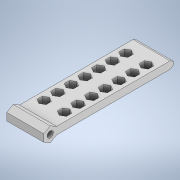
# Autodesk Inventor part: HexFlipper
Saved by Autodesk Inventor 2020 (Build 240168000, 168)
## iProperties
Created: 2023-12-22
Part Number: HexFlipper
Material: Generic
Document SubType Name: Modeling
Designer: smz3rm
Density: 1 g/cm^3
Appearance: Default
FlipperRodLength: 63.072 mm
Author: smz3rm
Autodesk Inventor part; units mm, degrees
ref_plane "YZ Plane" through (0, 0, 0) normal (1, 0, 0) x (0, 1, 0)
ref_plane "XZ Plane" through (0, 0, 0) normal (0, 1, 0) x (-1, 0, 0)
ref_plane "XY Plane" through (0, 0, 0) normal (0, 0, 1) x (1, 0, 0)
sketch "Sketch1" plane through (0, 0, 0) normal (1, 0, 0) x (0, 1, 0)
  line L0 (2, 35) -> (-2, 35)
  line L1 (-2, 35) -> (-2, -35)
  line L2 (-2, -35) -> (2, -35)
  line L3 (2, -35) -> (2, 35)
  line L4 (2, 35) -> (-2, -35) construction
  line L5 (-2, 35) -> (2, -35) construction
  line L6 (-1, -35) -> (-2, -33.2679)
  line L7 (-2, -33.2679) -> (-1, -31.5359)
  line L8 (-1, -31.5359) -> (1, -31.5359)
  line L9 (1, -31.5359) -> (2, -33.2679)
  line L10 (2, -33.2679) -> (1, -35)
  line L11 (1, -35) -> (-1, -35)
  line L12 (4, 31.5359) -> (2, 28.0718)
  line L13 (2, 28.0718) -> (-2, 28.0718)
  line L14 (-2, 28.0718) -> (-4, 31.5359)
  line L15 (-4, 31.5359) -> (-2, 35)
  line L16 (-2, 35) -> (2, 35)
  line L17 (2, 35) -> (4, 31.5359)
  circle A0 centre (0, 31.5359) radius 1.65
  point P0 (0, 0)
  point P1 (0, -33.2679)
  dimension "d0" = 4
  dimension "d1" = 70
  dimension "d2" = 3.3
  constraints: 36 end point, 4 point on line, 2 midpoint, 2 parallel, 1 centre point, 1 coincident, 1 horizontal, 1 perpendicular, 26 other
  measures "d0" distance of L2.end L1.end
  measures "d1" distance of L1.end L0.end
  measures "d2" diameter of A0
extrude "Extrusion1" add sketch "Sketch1" along normal mid plane 20 contours L3 L13 L1 L0 | L17 L12 L3 | L1 L14 L15 | L3 L9 L8 L7 L1 L13 | L10 L2 L6 L7 L8 L9
ref_plane "Work Plane1" through (-10, 2, 28.0718) normal (0, 0, -1) x (1, 0, 0)
sketch "Sketch2" plane through (-10, -1, -35) normal (0, 0, -1) x (-1, 0, 0)
  line L0 (-20, 2) -> (0, 2) projected
  line L1 (0, 0) -> (-20, 0) projected
  line L2 (-10, 2) -> (-10, 0)
  circle A0 centre (-10, 1) radius 1
  point P0 (-10, 1)
  dimension "d5" = 2
  constraints: 3 midpoint, 2 end point, 1 centre point, 1 vertical
  measures "d5" diameter of A0
extrude "Extrusion2" cut sketch "Sketch2" against normal up to surface (63.0718 mm away)
sketch "Sketch3" plane through (-10, 2, 28.0718) normal (0, 1, 0) x (1, 0, 0)
  line L0 (9, 63.0718) -> (9, 0) projected
  line L1 (11, 63.0718) -> (11, 0) projected
  line L2 (0, 0) -> (0, 61.3397) projected
  line L3 (0, 0) -> (20, 0) projected
  line L4 (20, 61.3397) -> (20, 0) projected
  line L5 (0, 61.3397) -> (20, 61.3397) projected
  line L6 (2, 2) -> (2, 59.3397)
  line L7 (2, 59.3397) -> (18, 59.3397)
  line L8 (18, 59.3397) -> (18, 2)
  line L9 (18, 2) -> (2, 2)
  line L10 (7, 63.0718) -> (7, 0)
  line L11 (13, 63.0718) -> (13, 0)
  line L12 (2, 51.5924) -> (2, 54.4791)
  line L13 (2, 54.4791) -> (4.5, 55.9225)
  line L14 (4.5, 55.9225) -> (7, 54.4791)
  line L15 (7, 54.4791) -> (7, 51.5924)
  line L16 (7, 51.5924) -> (4.5, 50.149)
  line L17 (4.5, 50.149) -> (2, 51.5924)
  line L18 (4.5, 42.7755) -> (2, 44.2189)
  line L19 (7, 44.2189) -> (4.5, 42.7755)
  line L20 (2, 47.1056) -> (4.5, 48.549)
  line L21 (4.5, 48.549) -> (7, 47.1056)
  line L22 (4.5, 35.402) -> (2, 36.8454)
  line L23 (7, 36.8454) -> (4.5, 35.402)
  line L24 (2, 39.7321) -> (4.5, 41.1755)
  line L25 (4.5, 41.1755) -> (7, 39.7321)
  line L26 (4.5, 28.0285) -> (2, 29.4719)
  line L27 (7, 29.4719) -> (4.5, 28.0285)
  line L28 (2, 32.3586) -> (4.5, 33.802)
  line L29 (4.5, 33.802) -> (7, 32.3586)
  line L30 (4.5, 20.655) -> (2, 22.0984)
  line L31 (7, 22.0984) -> (4.5, 20.655)
  line L32 (2, 24.9851) -> (4.5, 26.4285)
  line L33 (4.5, 26.4285) -> (7, 24.9851)
  line L34 (4.5, 13.2815) -> (2, 14.7249)
  line L35 (7, 14.7249) -> (4.5, 13.2815)
  line L36 (2, 17.6116) -> (4.5, 19.055)
  line L37 (4.5, 19.055) -> (7, 17.6116)
  line L38 (15.5, 55.9225) -> (18, 54.4791)
  line L39 (18, 54.4791) -> (18, 51.5924)
  line L40 (18, 51.5924) -> (15.5, 50.149)
  line L41 (15.5, 50.149) -> (13, 51.5924)
  line L42 (13, 51.5924) -> (13, 54.4791)
  line L43 (13, 54.4791) -> (15.5, 55.9225)
  line L44 (15.5, 42.7755) -> (13, 44.2189)
  line L45 (18, 44.2189) -> (15.5, 42.7755)
  line L46 (13, 47.1056) -> (15.5, 48.549)
  line L47 (15.5, 48.549) -> (18, 47.1056)
  line L48 (15.5, 35.402) -> (13, 36.8454)
  line L49 (18, 36.8454) -> (15.5, 35.402)
  line L50 (13, 39.7321) -> (15.5, 41.1755)
  line L51 (15.5, 41.1755) -> (18, 39.7321)
  line L52 (15.5, 28.0285) -> (13, 29.4719)
  line L53 (18, 29.4719) -> (15.5, 28.0285)
  line L54 (13, 32.3586) -> (15.5, 33.802)
  line L55 (15.5, 33.802) -> (18, 32.3586)
  line L56 (15.5, 20.655) -> (13, 22.0984)
  line L57 (18, 22.0984) -> (15.5, 20.655)
  line L58 (13, 24.9851) -> (15.5, 26.4285)
  line L59 (15.5, 26.4285) -> (18, 24.9851)
  line L60 (15.5, 13.2815) -> (13, 14.7249)
  line L61 (18, 14.7249) -> (15.5, 13.2815)
  line L62 (13, 17.6116) -> (15.5, 19.055)
  line L63 (15.5, 19.055) -> (18, 17.6116)
  line L64 (15.5, 5.908) -> (13, 7.3514)
  line L65 (18, 7.3514) -> (15.5, 5.908)
  line L66 (13, 10.2381) -> (15.5, 11.6815)
  line L67 (15.5, 11.6815) -> (18, 10.2381)
  line L68 (15.5, -1.4655) -> (13, -0.0221)
  line L69 (18, -0.0221) -> (15.5, -1.4655)
  line L70 (13, 2.8646) -> (15.5, 4.308)
  line L71 (15.5, 4.308) -> (18, 2.8646)
  line L72 (4.5, 5.908) -> (2, 7.3514)
  line L73 (7, 7.3514) -> (4.5, 5.908)
  line L74 (2, 10.2381) -> (4.5, 11.6815)
  line L75 (4.5, 11.6815) -> (7, 10.2381)
  line L76 (4.5, -1.4655) -> (2, -0.0221)
  line L77 (7, -0.0221) -> (4.5, -1.4655)
  line L78 (2, 2.8646) -> (4.5, 4.308)
  line L79 (4.5, 4.308) -> (7, 2.8646)
  line L80 (15.5, -8.839) -> (13, -7.3956)
  line L81 (18, -7.3956) -> (15.5, -8.839)
  line L82 (13, -4.5089) -> (15.5, -3.0655)
  line L83 (15.5, -3.0655) -> (18, -4.5089)
  line L84 (4.5, -8.839) -> (2, -7.3956)
  line L85 (7, -7.3956) -> (4.5, -8.839)
  line L86 (2, -4.5089) -> (4.5, -3.0655)
  line L87 (4.5, -3.0655) -> (7, -4.5089)
  line L88 (15.5, -16.2125) -> (13, -14.7691)
  line L89 (18, -14.7691) -> (15.5, -16.2125)
  line L90 (13, -11.8824) -> (15.5, -10.439)
  line L91 (15.5, -10.439) -> (18, -11.8824)
  line L92 (4.5, -16.2125) -> (2, -14.7691)
  line L93 (7, -14.7691) -> (4.5, -16.2125)
  line L94 (2, -11.8824) -> (4.5, -10.439)
  line L95 (4.5, -10.439) -> (7, -11.8824)
  line L96 (4.5, 53.0358) -> (15.5, 53.0358)
  point P0 (10, 28.0718)
  point P1 (18, 54.4791)
  point P2 (7, 54.4791)
  point P3 (18, 47.1056)
  point P4 (13, 47.1056)
  point P5 (13, 44.2189)
  point P6 (18, 44.2189)
  point P7 (7, 47.1056)
  point P8 (2, 47.1056)
  point P9 (2, 44.2189)
  point P10 (7, 44.2189)
  point P11 (18, 39.7321)
  point P12 (13, 39.7321)
  point P13 (13, 36.8454)
  point P14 (18, 36.8454)
  point P15 (7, 39.7321)
  point P16 (2, 39.7321)
  point P17 (2, 36.8454)
  point P18 (7, 36.8454)
  point P19 (18, 32.3586)
  point P20 (13, 32.3586)
  point P21 (13, 29.4719)
  point P22 (18, 29.4719)
  point P23 (7, 32.3586)
  point P24 (2, 32.3586)
  point P25 (2, 29.4719)
  point P26 (7, 29.4719)
  point P27 (18, 24.9851)
  point P28 (13, 24.9851)
  point P29 (13, 22.0984)
  point P30 (18, 22.0984)
  point P31 (7, 24.9851)
  point P32 (2, 24.9851)
  point P33 (2, 22.0984)
  point P34 (7, 22.0984)
  point P35 (18, 17.6116)
  point P36 (13, 17.6116)
  point P37 (13, 14.7249)
  point P38 (18, 14.7249)
  point P39 (7, 17.6116)
  point P40 (2, 17.6116)
  point P41 (2, 14.7249)
  point P42 (7, 14.7249)
  point P43 (18, 10.2381)
  point P44 (13, 10.2381)
  point P45 (13, 7.3514)
  point P46 (18, 7.3514)
  point P47 (7, 10.2381)
  point P48 (2, 10.2381)
  point P49 (2, 7.3514)
  point P50 (7, 7.3514)
  point P51 (18, 2.8646)
  point P52 (13, 2.8646)
  point P53 (13, 0.0621)
  point P54 (15.4164, 2)
  point P55 (15.5836, 2)
  point P56 (18, 3.3951)
  point P57 (7, 2.8646)
  point P58 (2, 2.8646)
  point P59 (2, 2.7775)
  point P60 (3.3466, 2)
  point P61 (5.6534, 2)
  point P62 (7, 2.7775)
  point P63 (13, 2)
  point P64 (13, 59.3397)
  point P65 (7, 59.3397)
  point P66 (7, 2)
  dimension "d8" = 2
  dimension "d9" = 2
  dimension "d10" = 2
  dimension "d11" = 5.7735
  dimension "d14" = 7.3735
  dimension "d21" = 7.3735
  constraints: 182 end point, 6 point on line, 2 parallel, 2 vertical, 1 horizontal, 209 other
  measures "d8" distance between parallel lines of L2 L6
  measures "d9" distance between parallel lines of L0 L10
  measures "d10" distance between parallel lines of L1 L11
  measures "d11" distance of L13.end L16.end
  measures "d14" distance of L16.end L18.start
  measures "d21" distance of L40.end L44.start
extrude "Extrusion3" cut sketch "Sketch3" against normal up to surface (4 mm away) contours L10 L16 L17 L6 L13 L14 | L11 L43 L38 L8 L40 L41 | L10 L19 L18 L6 L20 L21 | L73 L72 L6 L74 L75 L10 | L46 L47 L8 L45 L44 L11 | L11 L66 L67 L8 L65 L64 | L10 L23 L22 L6 L24 L25 | L35 L34 L6 L36 L37 L10 | L50 L51 L8 L49 L48 L11 | L11 L62 L63 L8 L61 L60 | L10 L27 L26 L6 L28 L29 | L31 L30 L6 L32 L33 L10 | L54 L55 L8 L53 L52 L11 | L11 L58 L59 L8 L57 L56
sketch "Sketch4" plane through (-10, 2, 28.0718) normal (0, 1, 0) x (1, 0, 0)
  line L0 (11, 63.0718) -> (11, 0) projected
  line L1 (9, 63.0718) -> (9, 0) projected
  point P0 (10, 28.0718)
  dimension "d28" = 63.0718
  measures "d28" distance of L1.start L1.end
equation "\"d0\" = FlipperThickness"
equation "\"d1\" = FlipperLength"
equation "\"d3\" = FlipperWidth"
equation "\"d5\" = FlipperRodDia"
equation "\"d6\" = FlipperWidth"
equation "\"d8\" = HexOffset"
equation "\"d9\" = HexOffset"
equation "\"d10\" = HexOffset"
equation "\"d14\" = d11 + HexSpacing"
equation "\"d21\" = d11 + HexSpacing"
equation "\"HexOffset\" = 2"
equation "\"HexSpacing\" = 1.6"
equation "\"FlipperRodLength\" = d28"
equation "\"FlipperThickness\" = 4"
equation "\"FlipperLength\" = 70"
equation "\"FlipperWidth\" = 20"
equation "\"FlipperRodDia\" = 2"
body "Solid1"
